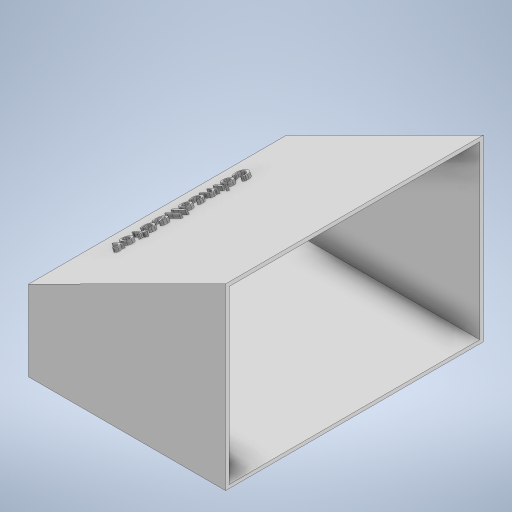
# Autodesk Inventor part: Part3
Saved by Autodesk Inventor 2023 (Build 270158030, 158C)
## iProperties
Created: 2023-04-28
Part Number: Part3
Material: Generic
Document SubType Name: Modeling
Designer: 22165
Density: 1 g/cm^3
Appearance: Default
Author: 22165
Autodesk Inventor part; units mm, degrees
ref_plane "YZ Plane" through (0, 0, 0) normal (1, 0, 0) x (0, 1, 0)
ref_plane "XZ Plane" through (0, 0, 0) normal (0, 1, 0) x (-1, 0, 0)
ref_plane "XY Plane" through (0, 0, 0) normal (0, 0, 1) x (1, 0, 0)
sketch "Sketch1" plane through (0, 0, 0) normal (0, 0, 1) x (1, 0, 0)
  line L0 (0, 0) -> (110, 0)
  line L1 (110, 0) -> (110, -100)
  line L2 (110, -100) -> (0, -100)
  line L3 (0, -100) -> (0, -55.0625)
  line L4 (110, 0) -> (0, -55.0625)
  dimension "d0" = 110
  dimension "d1" = 100
  dimension "d2" = 110
  dimension "d3" = 63.409
  dimension "d4" = 116.591
  dimension "d5" = 90
  constraints: 10 end point, 2 parallel, 1 horizontal, 1 perpendicular
  measures "d0" distance of L1.end L2.end
  measures "d1" distance of L0.end L1.end
  measures "d2" distance between parallel lines of L1 L3
  measures "d3" angle of L1 L4
  measures "d4" angle of L4 L3
  measures "d5" angle of L0 L1
extrude "Extrusion1" add sketch "Sketch1" along normal blind 144
shell "Shell2" thickness 2 removed faces 1 at (110, -66.6667, 48)
sketch "Sketch2" plane through (0, -55.0625, 144) normal (-0.4476, 0.8942, 0) x (0.8942, 0.4476, 0)
  line L0 (24.5895, 107) -> (24.5895, 52) construction
  line L1 (24.5895, 52) -> (21.4212, 52) construction
  line L2 (21.4212, 52) -> (21.4212, 107) construction
  line L3 (21.4212, 107) -> (24.5895, 107) construction
  line L4 (122.0106, 142) -> (1.2354, 142) projected
  line L5 (122.0106, 2) -> (1.2354, 2) projected
  spline S0 degree 2 poles (21.5723, 100.1724) (21.5723, 100.569) (22.0378, 100.7672) knots 0 0 0 1 1 1
  spline S1 degree 2 poles (22.0378, 100.7672) (22.4343, 100.9397) (22.5205, 101.0862) knots 0 0 0 1 1 1
  spline S2 degree 2 poles (22.5205, 101.0862) (22.5895, 101.2155) (22.5895, 101.7328) knots 0 0 0 1 1 1
  spline S3 degree 2 poles (22.5895, 101.7328) (22.5895, 102.6293) (21.2188, 103.7241) knots 0 0 0 1 1 1
  spline S4 degree 2 poles (21.2188, 103.7241) (19.374, 105.2069) (17.7274, 105.2069) knots 0 0 0 1 1 1
  spline S5 degree 2 poles (17.7274, 105.2069) (16.9257, 105.2069) (16.3567, 104.6897) knots 0 0 0 1 1 1
  spline S6 degree 2 poles (16.3567, 104.6897) (15.7619, 104.1638) (15.7619, 103.4224) knots 0 0 0 1 1 1
  spline S7 degree 2 poles (15.7619, 103.4224) (15.7619, 102.7845) (16.0895, 102.1466) knots 0 0 0 1 1 1
  spline S8 degree 2 poles (16.0895, 102.1466) (16.2791, 101.7845) (16.8223, 101.0431) knots 0 0 0 1 1 1
  spline S9 degree 2 poles (16.8223, 101.0431) (17.0809, 100.6897) (17.0809, 100.5086) knots 0 0 0 1 1 1
  spline S10 degree 2 poles (17.0809, 100.5086) (17.0809, 100.25) (16.6757, 99.8879) (16.4343, 99.8879) knots 0 0 0 1 2 2 2
  spline S11 degree 2 poles (16.4343, 99.8879) (16.1498, 99.8879) (15.9429, 100.1207) knots 0 0 0 1 1 1
  spline S12 degree 2 poles (15.9429, 100.1207) (14.4947, 101.7586) (14.4947, 103.4224) knots 0 0 0 1 1 1
  spline S13 degree 2 poles (14.4947, 103.4224) (14.4947, 104.7069) (15.4774, 105.5862) knots 0 0 0 1 1 1
  spline S14 degree 2 poles (15.4774, 105.5862) (16.4257, 106.4397) (17.7274, 106.4397) knots 0 0 0 1 1 1
  spline S15 degree 2 poles (17.7274, 106.4397) (19.8223, 106.4397) (22.0205, 104.681) knots 0 0 0 1 1 1
  spline S16 degree 2 poles (22.0205, 104.681) (23.8567, 103.2155) (23.8567, 101.7328) knots 0 0 0 1 1 1
  spline S17 degree 2 poles (23.8567, 101.7328) (23.8567, 101.431) (23.805, 100.9483) (23.736, 100.7586) knots 0 0 0 1 2 2 2
  spline S18 degree 2 poles (23.736, 100.7586) (24.055, 100.5431) (24.055, 100.1983) knots 0 0 0 1 1 1
  spline S19 degree 2 poles (24.055, 100.1983) (24.055, 99.7672) (23.4947, 99.6552) knots 0 0 0 1 1 1
  spline S20 degree 2 poles (23.4947, 99.6552) (22.986, 99.5603) (22.2619, 99.5603) knots 0 0 0 1 1 1
  spline S21 degree 2 poles (22.2619, 99.5603) (22.0033, 99.5603) (21.8136, 99.6983) knots 0 0 0 1 1 1
  spline S22 degree 2 poles (21.8136, 99.6983) (21.5723, 99.8621) (21.5723, 100.1724) knots 0 0 0 1 1 1
  spline S23 degree 2 poles (14.2791, 96.181) (14.2791, 97.2155) (15.0464, 97.9655) knots 0 0 0 1 1 1
  spline S24 degree 2 poles (15.0464, 97.9655) (15.8998, 98.8017) (17.3395, 98.8448) knots 0 0 0 1 1 1
  spline S25 degree 2 poles (17.3395, 98.8448) (18.736, 98.8793) (19.7964, 98.1379) knots 0 0 0 1 1 1
  spline S26 degree 2 poles (19.7964, 98.1379) (21.055, 97.2759) (21.055, 95.7328) knots 0 0 0 1 1 1
  spline S27 degree 2 poles (21.055, 95.7328) (21.055, 94.4914) (19.9257, 93.8621) knots 0 0 0 1 1 1
  spline S28 degree 2 poles (19.9257, 93.8621) (19.0119, 93.3534) (17.7188, 93.3707) knots 0 0 0 1 1 1
  spline S29 degree 2 poles (17.7188, 93.3707) (16.3481, 93.3879) (15.3826, 94.0862) knots 0 0 0 1 1 1
  spline S30 degree 2 poles (15.3826, 94.0862) (14.2791, 94.8793) (14.2791, 96.181) knots 0 0 0 1 1 1
  spline S31 degree 2 poles (19.7964, 95.8103) (19.805, 96.7155) (18.9343, 97.2241) knots 0 0 0 1 1 1
  spline S32 degree 2 poles (18.9343, 97.2241) (18.236, 97.6293) (17.3395, 97.6293) knots 0 0 0 1 1 1
  spline S33 degree 2 poles (17.3395, 97.6293) (16.4429, 97.6293) (15.9429, 97.1379) knots 0 0 0 1 1 1
  spline S34 degree 2 poles (15.9429, 97.1379) (15.5291, 96.7328) (15.5291, 96.181) knots 0 0 0 1 1 1
  spline S35 degree 2 poles (15.5291, 96.181) (15.5291, 95.5345) (15.9947, 95.0776) knots 0 0 0 1 1 1
  spline S36 degree 2 poles (15.9947, 95.0776) (16.5205, 94.5517) (17.3998, 94.5172) knots 0 0 0 1 1 1
  spline S37 degree 2 poles (17.3998, 94.5172) (19.7878, 94.431) (19.7964, 95.8103) knots 0 0 0 1 1 1
  spline S38 degree 2 poles (17.4516, 90.3879) (17.0809, 90.3879) (15.5981, 90.3448) (15.2274, 90.3448) knots 0 0 0 1 2 2 2
  spline S39 degree 2 poles (15.2274, 90.3448) (14.9516, 90.3448) (14.6067, 90.681) (14.6067, 90.9483) knots 0 0 0 1 2 2 2
  spline S40 degree 2 poles (14.6067, 90.9483) (14.6067, 91.2155) (14.9516, 91.5603) (15.2274, 91.5603) knots 0 0 0 1 2 2 2
  spline S41 degree 2 poles (15.2274, 91.5603) (15.5981, 91.5603) (17.0809, 91.6034) (17.4516, 91.6034) knots 0 0 0 1 2 2 2
  spline S42 degree 2 poles (17.4516, 91.6034) (18.0291, 91.6034) (19.7705, 91.4828) (20.3481, 91.4828) knots 0 0 0 1 2 2 2
  spline S43 degree 2 poles (20.3481, 91.4828) (20.6326, 91.4828) (20.9774, 91.1379) (20.9774, 90.8707) knots 0 0 0 1 2 2 2
  spline S44 degree 2 poles (20.9774, 90.8707) (20.9774, 90.6121) (20.6326, 90.2672) (20.3481, 90.2672) knots 0 0 0 1 2 2 2
  spline S45 degree 2 poles (20.3481, 90.2672) (19.7705, 90.2672) (18.0291, 90.3879) (17.4516, 90.3879) knots 0 0 0 1 2 2 2
  spline S46 degree 2 poles (22.4774, 90.6724) (22.4774, 90.9741) (22.8998, 91.4052) (23.1929, 91.4052) knots 0 0 0 1 2 2 2
  spline S47 degree 2 poles (23.1929, 91.4052) (23.486, 91.4052) (23.9085, 90.9741) (23.9085, 90.6724) knots 0 0 0 1 2 2 2
  spline S48 degree 2 poles (23.9085, 90.6724) (23.9085, 90.3793) (23.486, 89.9483) (23.1929, 89.9483) knots 0 0 0 1 2 2 2
  spline S49 degree 2 poles (23.1929, 89.9483) (22.8998, 89.9483) (22.4774, 90.3793) (22.4774, 90.6724) knots 0 0 0 1 2 2 2
  spline S50 degree 2 poles (14.2016, 83.5517) (14.2016, 84.0776) (14.7791, 84.1466) knots 0 0 0 1 1 1
  line L6 (14.7791, 84.1466) -> (16.1412, 84.319)
  spline S51 degree 2 poles (16.1412, 84.319) (16.8654, 84.4052) (17.4947, 84.4052) knots 0 0 0 1 1 1
  spline S52 degree 2 poles (17.4947, 84.4052) (17.6671, 84.4052) (18.4947, 84.3621) (18.6671, 84.3621) knots 0 0 0 1 2 2 2
  spline S53 degree 2 poles (18.6671, 84.3621) (20.0033, 84.3621) (20.0033, 84.8534) knots 0 0 0 1 1 1
  spline S54 degree 2 poles (20.0033, 84.8534) (20.0033, 85.5517) (19.1843, 86.181) knots 0 0 0 1 1 1
  spline S55 degree 2 poles (19.1843, 86.181) (18.4343, 86.75) (17.2878, 87.069) knots 0 0 0 1 1 1
  spline S56 degree 2 poles (17.2878, 87.069) (17.0464, 87.0862) (16.6843, 87.1293) knots 0 0 0 1 1 1
  spline S57 degree 2 poles (16.6843, 87.1293) (16.374, 87.1638) (16.0809, 87.1638) knots 0 0 0 1 1 1
  spline S58 degree 2 poles (16.0809, 87.1638) (15.8998, 87.1638) (15.1585, 87.0862) (14.9688, 87.0862) knots 0 0 0 1 2 2 2
  spline S59 degree 2 poles (14.9688, 87.0862) (14.6929, 87.0862) (14.3481, 87.431) (14.3481, 87.6983) knots 0 0 0 1 2 2 2
  spline S60 degree 2 poles (14.3481, 87.6983) (14.3481, 87.9655) (14.6929, 88.3017) (14.9688, 88.3017) knots 0 0 0 1 2 2 2
  spline S61 degree 2 poles (14.9688, 88.3017) (15.1585, 88.3017) (15.8998, 88.3793) (16.0895, 88.3793) knots 0 0 0 1 2 2 2
  spline S62 degree 2 poles (16.0895, 88.3793) (16.7274, 88.3793) (18.9774, 88.2069) (19.6154, 88.2069) knots 0 0 0 1 2 2 2
  spline S63 degree 2 poles (19.6154, 88.2069) (19.8136, 88.2069) (20.5981, 88.25) (20.7964, 88.25) knots 0 0 0 1 2 2 2
  spline S64 degree 2 poles (20.7964, 88.25) (21.0636, 88.25) (21.3998, 87.8966) (21.3998, 87.6379) knots 0 0 0 1 2 2 2
  spline S65 degree 2 poles (21.3998, 87.6379) (21.3998, 87.069) (20.5895, 87.0086) knots 0 0 0 1 1 1
  line L7 (20.5895, 87.0086) -> (19.8654, 86.9914)
  spline S66 degree 2 poles (19.8654, 86.9914) (21.2533, 85.9569) (21.2533, 84.8621) knots 0 0 0 1 1 1
  spline S67 degree 2 poles (21.2533, 84.8621) (21.2533, 83.8707) (20.3826, 83.4828) knots 0 0 0 1 1 1
  spline S68 degree 2 poles (20.3826, 83.4828) (19.7964, 83.2155) (18.6585, 83.1897) knots 0 0 0 1 1 1
  line L8 (18.6585, 83.1897) -> (18.0378, 83.1897)
  line L9 (18.0378, 83.1897) -> (17.4602, 83.1983)
  spline S69 degree 2 poles (17.4602, 83.1983) (16.9516, 83.1983) (15.3223, 82.931) (14.8136, 82.931) knots 0 0 0 1 2 2 2
  spline S70 degree 2 poles (14.8136, 82.931) (14.5378, 82.931) (14.2016, 83.2845) (14.2016, 83.5517) knots 0 0 0 1 2 2 2
  spline S71 degree 2 poles (14.2533, 78.8707) (14.2533, 80.1379) (15.0205, 80.9914) knots 0 0 0 1 1 1
  spline S72 degree 2 poles (15.0205, 80.9914) (15.8223, 81.8793) (17.1412, 81.8793) knots 0 0 0 1 1 1
  spline S73 degree 2 poles (17.1412, 81.8793) (18.3912, 81.8793) (19.7274, 81.0431) knots 0 0 0 1 1 1
  spline S74 degree 2 poles (19.7274, 81.0431) (21.2102, 80.1207) (21.2102, 78.9569) knots 0 0 0 1 1 1
  spline S75 degree 2 poles (21.2102, 78.9569) (21.2102, 78.3448) (20.9257, 77.6034) knots 0 0 0 1 1 1
  spline S76 degree 2 poles (20.9257, 77.6034) (20.5636, 76.6552) (20.0378, 76.6552) knots 0 0 0 1 1 1
  spline S77 degree 2 poles (20.0378, 76.6552) (19.7964, 76.6552) (19.4343, 76.9655) (19.4343, 77.1897) knots 0 0 0 1 2 2 2
  spline S78 degree 2 poles (19.4343, 77.1897) (19.4343, 77.3707) (19.6498, 77.6379) (19.7533, 77.7586) knots 0 0 0 1 2 2 2
  spline S79 degree 2 poles (19.7533, 77.7586) (20.0464, 78.1293) (20.0464, 78.9569) knots 0 0 0 1 1 1
  spline S80 degree 2 poles (20.0464, 78.9569) (20.0464, 79.5862) (18.9257, 80.2069) knots 0 0 0 1 1 1
  spline S81 degree 2 poles (18.9257, 80.2069) (17.8912, 80.7672) (17.1412, 80.7672) knots 0 0 0 1 1 1
  spline S82 degree 2 poles (17.1412, 80.7672) (16.3223, 80.7672) (15.8567, 80.2069) knots 0 0 0 1 1 1
  spline S83 degree 2 poles (15.8567, 80.2069) (15.4171, 79.6897) (15.4171, 78.8707) knots 0 0 0 1 1 1
  spline S84 degree 2 poles (15.4171, 78.8707) (15.4171, 78.5) (15.6154, 78.0776) knots 0 0 0 1 1 1
  line L10 (15.6154, 78.0776) -> (16.0033, 77.3621)
  spline S85 degree 2 poles (16.0033, 77.3621) (16.0981, 77.181) (16.0981, 77.0948) knots 0 0 0 1 1 1
  spline S86 degree 2 poles (16.0981, 77.0948) (16.0981, 76.8707) (15.736, 76.5345) (15.4947, 76.5345) knots 0 0 0 1 2 2 2
  spline S87 degree 2 poles (15.4947, 76.5345) (15.0464, 76.5345) (14.624, 77.4914) knots 0 0 0 1 1 1
  spline S88 degree 2 poles (14.624, 77.4914) (14.2533, 78.319) (14.2533, 78.8707) knots 0 0 0 1 1 1
  spline S89 degree 2 poles (14.2791, 72.8276) (14.2791, 73.8621) (15.0464, 74.6121) knots 0 0 0 1 1 1
  spline S90 degree 2 poles (15.0464, 74.6121) (15.8998, 75.4483) (17.3395, 75.4914) knots 0 0 0 1 1 1
  spline S91 degree 2 poles (17.3395, 75.4914) (18.736, 75.5259) (19.7964, 74.7845) knots 0 0 0 1 1 1
  spline S92 degree 2 poles (19.7964, 74.7845) (21.055, 73.9224) (21.055, 72.3793) knots 0 0 0 1 1 1
  spline S93 degree 2 poles (21.055, 72.3793) (21.055, 71.1379) (19.9257, 70.5086) knots 0 0 0 1 1 1
  spline S94 degree 2 poles (19.9257, 70.5086) (19.0119, 70) (17.7188, 70.0172) knots 0 0 0 1 1 1
  spline S95 degree 2 poles (17.7188, 70.0172) (16.3481, 70.0345) (15.3826, 70.7328) knots 0 0 0 1 1 1
  spline S96 degree 2 poles (15.3826, 70.7328) (14.2791, 71.5259) (14.2791, 72.8276) knots 0 0 0 1 1 1
  spline S97 degree 2 poles (19.7964, 72.4569) (19.805, 73.3621) (18.9343, 73.8707) knots 0 0 0 1 1 1
  spline S98 degree 2 poles (18.9343, 73.8707) (18.236, 74.2759) (17.3395, 74.2759) knots 0 0 0 1 1 1
  spline S99 degree 2 poles (17.3395, 74.2759) (16.4429, 74.2759) (15.9429, 73.7845) knots 0 0 0 1 1 1
  spline S100 degree 2 poles (15.9429, 73.7845) (15.5291, 73.3793) (15.5291, 72.8276) knots 0 0 0 1 1 1
  spline S101 degree 2 poles (15.5291, 72.8276) (15.5291, 72.181) (15.9947, 71.7241) knots 0 0 0 1 1 1
  spline S102 degree 2 poles (15.9947, 71.7241) (16.5205, 71.1983) (17.3998, 71.1638) knots 0 0 0 1 1 1
  spline S103 degree 2 poles (17.3998, 71.1638) (19.7878, 71.0776) (19.7964, 72.4569) knots 0 0 0 1 1 1
  line L11 (19.5033, 66.9224) -> (16.4257, 67.0086)
  spline S104 degree 2 poles (16.4257, 67.0086) (15.9343, 67.0086) (14.9947, 67.0603) knots 0 0 0 1 1 1
  spline S105 degree 2 poles (14.9947, 67.0603) (14.374, 67.1207) (14.374, 67.6638) knots 0 0 0 1 1 1
  spline S106 degree 2 poles (14.374, 67.6638) (14.374, 68.2759) (15.0033, 68.2759) knots 0 0 0 1 1 1
  spline S107 degree 2 poles (15.0033, 68.2759) (15.7533, 68.2759) (18.7533, 68.1379) (19.5033, 68.1379) knots 0 0 0 1 2 2 2
  spline S108 degree 2 poles (19.5033, 68.1379) (20.4774, 68.1379) (22.9947, 68.0776) (23.9688, 68.0776) knots 0 0 0 1 2 2 2
  spline S109 degree 2 poles (23.9688, 68.0776) (24.5895, 68.0776) (24.5895, 67.4741) knots 0 0 0 1 1 1
  spline S110 degree 2 poles (24.5895, 67.4741) (24.5895, 66.8621) (23.9688, 66.8621) knots 0 0 0 1 1 1
  spline S111 degree 2 poles (23.9688, 66.8621) (22.9947, 66.8621) (20.4774, 66.9224) (19.5033, 66.9224) knots 0 0 0 1 2 2 2
  line L12 (19.5033, 63.4569) -> (16.4257, 63.5431)
  spline S112 degree 2 poles (16.4257, 63.5431) (15.9343, 63.5431) (14.9947, 63.5948) knots 0 0 0 1 1 1
  spline S113 degree 2 poles (14.9947, 63.5948) (14.374, 63.6552) (14.374, 64.1983) knots 0 0 0 1 1 1
  spline S114 degree 2 poles (14.374, 64.1983) (14.374, 64.8103) (15.0033, 64.8103) knots 0 0 0 1 1 1
  spline S115 degree 2 poles (15.0033, 64.8103) (15.7533, 64.8103) (18.7533, 64.6724) (19.5033, 64.6724) knots 0 0 0 1 2 2 2
  spline S116 degree 2 poles (19.5033, 64.6724) (20.4774, 64.6724) (22.9947, 64.6121) (23.9688, 64.6121) knots 0 0 0 1 2 2 2
  spline S117 degree 2 poles (23.9688, 64.6121) (24.5895, 64.6121) (24.5895, 64.0086) knots 0 0 0 1 1 1
  spline S118 degree 2 poles (24.5895, 64.0086) (24.5895, 63.3966) (23.9688, 63.3966) knots 0 0 0 1 1 1
  spline S119 degree 2 poles (23.9688, 63.3966) (22.9947, 63.3966) (20.4774, 63.4569) (19.5033, 63.4569) knots 0 0 0 1 2 2 2
  spline S120 degree 2 poles (14.3567, 58.681) (14.3567, 60.0776) (15.055, 60.9397) knots 0 0 0 1 1 1
  spline S121 degree 2 poles (15.055, 60.9397) (15.8309, 61.8879) (17.2188, 61.8879) knots 0 0 0 1 1 1
  spline S122 degree 2 poles (17.2188, 61.8879) (18.8309, 61.8879) (19.9171, 61.1121) knots 0 0 0 1 1 1
  spline S123 degree 2 poles (19.9171, 61.1121) (21.1067, 60.2586) (21.1067, 58.8448) knots 0 0 0 1 1 1
  spline S124 degree 2 poles (21.1067, 58.8448) (21.1067, 57.819) (20.7619, 57.1724) knots 0 0 0 1 1 1
  spline S125 degree 2 poles (20.7619, 57.1724) (20.3309, 56.3707) (19.4516, 56.3707) knots 0 0 0 1 1 1
  spline S126 degree 2 poles (19.4516, 56.3707) (18.8309, 56.3707) (18.3223, 57.069) knots 0 0 0 1 1 1
  spline S127 degree 2 poles (18.3223, 57.069) (18.0981, 57.3793) (17.6326, 58.3793) knots 0 0 0 1 1 1
  line L13 (17.6326, 58.3793) -> (16.5119, 60.7414)
  spline S128 degree 2 poles (16.5119, 60.7414) (15.9947, 60.3966) (15.4774, 59.3621) (15.4774, 58.681) knots 0 0 0 1 2 2 2
  spline S129 degree 2 poles (15.4774, 58.681) (15.4774, 58.25) (15.6412, 57.681) knots 0 0 0 1 1 1
  spline S130 degree 2 poles (15.6412, 57.681) (15.8395, 56.9483) (16.5033, 56.5259) (16.5033, 56.2845) knots 0 0 0 1 2 2 2
  spline S131 degree 2 poles (16.5033, 56.2845) (16.5033, 56.069) (16.1757, 55.7328) (15.9602, 55.7328) knots 0 0 0 1 2 2 2
  spline S132 degree 2 poles (15.9602, 55.7328) (15.2705, 55.7328) (14.7791, 56.8362) knots 0 0 0 1 1 1
  spline S133 degree 2 poles (14.7791, 56.8362) (14.3567, 57.7845) (14.3567, 58.681) knots 0 0 0 1 1 1
  spline S134 degree 2 poles (19.9947, 58.8448) (19.9947, 59.5948) (18.8223, 60.5948) (17.6498, 60.8448) knots 0 0 0 1 2 2 2
  line L14 (17.6498, 60.8448) -> (18.555, 58.9483)
  spline S135 degree 2 poles (18.555, 58.9483) (19.0981, 57.8276) (19.5033, 57.3534) knots 0 0 0 1 1 1
  spline S136 degree 2 poles (19.5033, 57.3534) (19.9947, 57.8879) (19.9947, 58.8448) knots 0 0 0 1 1 1
  spline S137 degree 2 poles (14.2533, 51.8276) (14.2533, 53.0948) (15.0205, 53.9483) knots 0 0 0 1 1 1
  spline S138 degree 2 poles (15.0205, 53.9483) (15.8223, 54.8362) (17.1412, 54.8362) knots 0 0 0 1 1 1
  spline S139 degree 2 poles (17.1412, 54.8362) (18.3912, 54.8362) (19.7274, 54) knots 0 0 0 1 1 1
  spline S140 degree 2 poles (19.7274, 54) (21.2102, 53.0776) (21.2102, 51.9138) knots 0 0 0 1 1 1
  spline S141 degree 2 poles (21.2102, 51.9138) (21.2102, 51.3017) (20.9257, 50.5603) knots 0 0 0 1 1 1
  spline S142 degree 2 poles (20.9257, 50.5603) (20.5636, 49.6121) (20.0378, 49.6121) knots 0 0 0 1 1 1
  spline S143 degree 2 poles (20.0378, 49.6121) (19.7964, 49.6121) (19.4343, 49.9224) (19.4343, 50.1466) knots 0 0 0 1 2 2 2
  spline S144 degree 2 poles (19.4343, 50.1466) (19.4343, 50.3276) (19.6498, 50.5948) (19.7533, 50.7155) knots 0 0 0 1 2 2 2
  spline S145 degree 2 poles (19.7533, 50.7155) (20.0464, 51.0862) (20.0464, 51.9138) knots 0 0 0 1 1 1
  spline S146 degree 2 poles (20.0464, 51.9138) (20.0464, 52.5431) (18.9257, 53.1638) knots 0 0 0 1 1 1
  spline S147 degree 2 poles (18.9257, 53.1638) (17.8912, 53.7241) (17.1412, 53.7241) knots 0 0 0 1 1 1
  spline S148 degree 2 poles (17.1412, 53.7241) (16.3223, 53.7241) (15.8567, 53.1638) knots 0 0 0 1 1 1
  spline S149 degree 2 poles (15.8567, 53.1638) (15.4171, 52.6466) (15.4171, 51.8276) knots 0 0 0 1 1 1
  spline S150 degree 2 poles (15.4171, 51.8276) (15.4171, 51.4569) (15.6154, 51.0345) knots 0 0 0 1 1 1
  line L15 (15.6154, 51.0345) -> (16.0033, 50.319)
  spline S151 degree 2 poles (16.0033, 50.319) (16.0981, 50.1379) (16.0981, 50.0517) knots 0 0 0 1 1 1
  spline S152 degree 2 poles (16.0981, 50.0517) (16.0981, 49.8276) (15.736, 49.4914) (15.4947, 49.4914) knots 0 0 0 1 2 2 2
  spline S153 degree 2 poles (15.4947, 49.4914) (15.0464, 49.4914) (14.624, 50.4483) knots 0 0 0 1 1 1
  spline S154 degree 2 poles (14.624, 50.4483) (14.2533, 51.2759) (14.2533, 51.8276) knots 0 0 0 1 1 1
  spline S155 degree 2 poles (19.9085, 43.9741) (19.9085, 44.1034) (19.9343, 44.4569) (19.9343, 44.5862) knots 0 0 0 1 2 2 2
  spline S156 degree 2 poles (19.9343, 44.5862) (19.9343, 44.7328) (19.8395, 45.431) knots 0 0 0 1 1 1
  line L16 (19.8395, 45.431) -> (16.1843, 45.319)
  line L17 (16.1843, 45.319) -> (15.9171, 45.3103)
  line L18 (15.9171, 45.3103) -> (15.5981, 45.3017)
  spline S157 degree 2 poles (15.5981, 45.3017) (14.2447, 45.2759) (14.2447, 45.9483) knots 0 0 0 1 1 1
  spline S158 degree 2 poles (14.2447, 45.9483) (14.2447, 46.1983) (14.5636, 46.5603) (14.805, 46.5603) knots 0 0 0 1 2 2 2
  spline S159 degree 2 poles (14.805, 46.5603) (15.0464, 46.5603) (15.986, 46.5259) (16.2188, 46.5259) knots 0 0 0 1 2 2 2
  line L19 (16.2188, 46.5259) -> (19.8309, 46.6466)
  spline S160 degree 2 poles (19.8309, 46.6466) (19.8481, 47.0948) (19.9343, 48.0172) knots 0 0 0 1 1 1
  spline S161 degree 2 poles (19.9343, 48.0172) (20.0119, 48.569) (20.5464, 48.569) knots 0 0 0 1 1 1
  spline S162 degree 2 poles (20.5464, 48.569) (20.8223, 48.569) (21.1757, 48.2328) (21.1757, 47.9741) knots 0 0 0 1 2 2 2
  line L20 (21.1757, 47.9741) -> (21.0723, 46.681)
  spline S163 degree 2 poles (21.0723, 46.681) (21.3912, 46.681) (22.4429, 46.7328) (22.6757, 46.7328) knots 0 0 0 1 2 2 2
  spline S164 degree 2 poles (22.6757, 46.7328) (22.9429, 46.7328) (23.2791, 46.3793) (23.2791, 46.1207) knots 0 0 0 1 2 2 2
  spline S165 degree 2 poles (23.2791, 46.1207) (23.2791, 45.5603) (22.374, 45.4655) knots 0 0 0 1 1 1
  spline S166 degree 2 poles (22.374, 45.4655) (22.1412, 45.4483) (21.8223, 45.4483) knots 0 0 0 1 1 1
  line L21 (21.8223, 45.4483) -> (21.4602, 45.4569)
  line L22 (21.4602, 45.4569) -> (21.0809, 45.4655)
  spline S167 degree 2 poles (21.0809, 45.4655) (21.1757, 44.6983) (21.1757, 44.5862) knots 0 0 0 1 1 1
  spline S168 degree 2 poles (21.1757, 44.5862) (21.1757, 43.9483) (21.1154, 43.75) knots 0 0 0 1 1 1
  spline S169 degree 2 poles (21.1154, 43.75) (20.9947, 43.3707) (20.5378, 43.3707) knots 0 0 0 1 1 1
  spline S170 degree 2 poles (20.5378, 43.3707) (20.2619, 43.3707) (19.9085, 43.7069) (19.9085, 43.9741) knots 0 0 0 1 2 2 2
  spline S171 degree 2 poles (14.2791, 39.819) (14.2791, 40.8534) (15.0464, 41.6034) knots 0 0 0 1 1 1
  spline S172 degree 2 poles (15.0464, 41.6034) (15.8998, 42.4397) (17.3395, 42.4828) knots 0 0 0 1 1 1
  spline S173 degree 2 poles (17.3395, 42.4828) (18.736, 42.5172) (19.7964, 41.7759) knots 0 0 0 1 1 1
  spline S174 degree 2 poles (19.7964, 41.7759) (21.055, 40.9138) (21.055, 39.3707) knots 0 0 0 1 1 1
  spline S175 degree 2 poles (21.055, 39.3707) (21.055, 38.1293) (19.9257, 37.5) knots 0 0 0 1 1 1
  spline S176 degree 2 poles (19.9257, 37.5) (19.0119, 36.9914) (17.7188, 37.0086) knots 0 0 0 1 1 1
  spline S177 degree 2 poles (17.7188, 37.0086) (16.3481, 37.0259) (15.3826, 37.7241) knots 0 0 0 1 1 1
  spline S178 degree 2 poles (15.3826, 37.7241) (14.2791, 38.5172) (14.2791, 39.819) knots 0 0 0 1 1 1
  spline S179 degree 2 poles (19.7964, 39.4483) (19.805, 40.3534) (18.9343, 40.8621) knots 0 0 0 1 1 1
  spline S180 degree 2 poles (18.9343, 40.8621) (18.236, 41.2672) (17.3395, 41.2672) knots 0 0 0 1 1 1
  spline S181 degree 2 poles (17.3395, 41.2672) (16.4429, 41.2672) (15.9429, 40.7759) knots 0 0 0 1 1 1
  spline S182 degree 2 poles (15.9429, 40.7759) (15.5291, 40.3707) (15.5291, 39.819) knots 0 0 0 1 1 1
  spline S183 degree 2 poles (15.5291, 39.819) (15.5291, 39.1724) (15.9947, 38.7155) knots 0 0 0 1 1 1
  spline S184 degree 2 poles (15.9947, 38.7155) (16.5205, 38.1897) (17.3998, 38.1552) knots 0 0 0 1 1 1
  spline S185 degree 2 poles (17.3998, 38.1552) (19.7878, 38.069) (19.7964, 39.4483) knots 0 0 0 1 1 1
  spline S186 degree 2 poles (19.2102, 30.6724) (18.4343, 30.7155) (18.4343, 31.2845) knots 0 0 0 1 1 1
  spline S187 degree 2 poles (18.4343, 31.2845) (18.4343, 31.819) (19.0464, 31.819) knots 0 0 0 1 1 1
  spline S188 degree 2 poles (19.0464, 31.819) (19.1671, 31.819) (19.486, 31.8362) knots 0 0 0 1 1 1
  line L23 (19.486, 31.8362) -> (20.0033, 31.8534)
  spline S189 degree 2 poles (20.0033, 31.8534) (19.8826, 32.8276) (19.4516, 33.4224) knots 0 0 0 1 1 1
  spline S190 degree 2 poles (19.4516, 33.4224) (19.055, 33.9741) (18.2447, 34.3362) knots 0 0 0 1 1 1
  line L24 (18.2447, 34.3362) -> (14.8481, 34.3276)
  spline S191 degree 2 poles (14.8481, 34.3276) (14.2274, 34.3276) (14.2274, 34.9397) knots 0 0 0 1 1 1
  spline S192 degree 2 poles (14.2274, 34.9397) (14.2274, 35.4828) (14.8481, 35.4828) knots 0 0 0 1 1 1
  line L25 (14.8481, 35.4828) -> (19.1929, 35.4828)
  spline S193 degree 2 poles (19.1929, 35.4828) (19.3912, 35.4828) (20.2102, 35.4483) (20.4171, 35.4483) knots 0 0 0 1 2 2 2
  spline S194 degree 2 poles (20.4171, 35.4483) (21.0378, 35.4483) (21.0378, 34.9052) knots 0 0 0 1 1 1
  spline S195 degree 2 poles (21.0378, 34.9052) (21.0378, 34.3017) (20.0119, 34.2931) knots 0 0 0 1 1 1
  spline S196 degree 2 poles (20.0119, 34.2931) (21.1585, 33.1034) (21.1585, 31.6552) knots 0 0 0 1 1 1
  spline S197 degree 2 poles (21.1585, 31.6552) (21.1585, 31.1552) (20.3998, 30.6638) (19.6412, 30.6638) knots 0 0 0 1 2 2 2
  spline S198 degree 2 poles (19.6412, 30.6638) (19.3223, 30.6638) (19.2102, 30.6724) knots 0 0 0 1 1 1
  point P0 (24.6471, 144)
  point P1 (23.0053, 107)
  point P2 (23.0053, 52)
  dimension "d10" = 35
  dimension "d11" = 50
  constraints: 2 midpoint, 2 other
  measures "d10" distance from line of L4 point (23.005, 107)
  measures "d11" distance from line of L5 point (23.005, 52)
extrude "Extrusion2" add sketch "Sketch2" along normal blind 2
body "Solid1"
